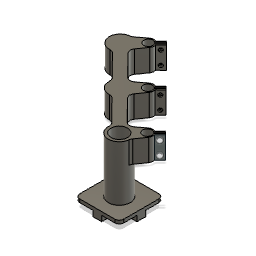
splicer_sample-fixation_004 (Autodesk Fusion 360 design; units mm, degrees)
Autodesk Fusion 360 part; units mm, degrees
sketch "Sketch1" plane through (0, 0, 0) normal (0, 1, 0) x (1, 0, 0)
  line L0 (20, -20) -> (-20, -20)
  line L1 (-20, -20) -> (-20, 20)
  line L2 (-20, 20) -> (20, 20)
  line L3 (20, 20) -> (20, -20)
  line L4 (20, -20) -> (-20, 20) construction
  line L5 (-20, -20) -> (20, 20) construction
  line L6 (-20, 4) -> (-15, 4)
  line L7 (-15, 4) -> (-15, -4)
  line L8 (-15, -4) -> (-20, -4)
  line L9 (-20, -4) -> (-20, 4)
  line L10 (-4, 20) -> (4, 20)
  line L11 (4, 20) -> (4, 15)
  line L12 (4, 15) -> (-4, 15)
  line L13 (-4, 15) -> (-4, 20)
  line L14 (20, 4) -> (15, 4)
  line L15 (15, 4) -> (15, -4)
  line L16 (15, -4) -> (20, -4)
  line L17 (20, -4) -> (20, 4)
  line L18 (-4, -20) -> (4, -20)
  line L19 (4, -20) -> (4, -15)
  line L20 (4, -15) -> (-4, -15)
  line L21 (-4, -15) -> (-4, -20)
  dimension "d1" = 40
  dimension "d2" = 40
  dimension "d3" = 5
  dimension "d4" = 8
  dimension "d5" = 16
  dimension "d6" = 5
  dimension "d7" = 16
  dimension "d8" = 8
  dimension "d9" = 5
  dimension "d10" = 5
  dimension "d11" = 8
  dimension "d12" = 8
  dimension "d13" = 16
  dimension "d14" = 16
  constraint horizontal L0
  constraint perpendicular L0 L1
  constraint parallel L0 L2
  constraint parallel L1 L3
  constraint coincident L4 origin
  constraint coincident L5 origin
  constraint horizontal L6
  constraint vertical L7
  constraint horizontal L8
  constraint vertical L9
  constraint coincident L1 L6.start
  constraint horizontal L10
  constraint vertical L11
  constraint horizontal L12
  constraint vertical L13
  constraint coincident L2 L10.start
  constraint horizontal L14
  constraint vertical L15
  constraint horizontal L16
  constraint vertical L17
  constraint coincident L3 L14.start
  constraint horizontal L18
  constraint vertical L19
  constraint horizontal L20
  constraint vertical L21
  constraint coincident L0 L18.start
  measures "d1" distance of L1.end L2.end
  measures "d2" distance of L0.end L1.end
  measures "d3" distance of L6.start L6.end
  measures "d4" distance of L6.start L8.end
  measures "d5" distance of L1.end L6.start
  measures "d6" distance of L10.start L12.end
  measures "d7" distance of L1.end L10.start
  measures "d8" distance of L11 L13
  measures "d9" distance of L18.start L20.end
  measures "d10" distance of L14.start L14.end
  measures "d11" distance of L14.end L15.end
  measures "d12" distance of L19.end L20.end
  measures "d13" distance of L1 L21
  measures "d14" distance of L0.start L16
extrude "Extrude1" add sketch "Sketch1" against normal blind 3 contours L0 L1 L2 L3 L6 L7 L8 L11 L12 L13 L14 L15 L16 L19 L20 L21 makes body 1
extrude "Extrude2" add sketch "Sketch1" against normal blind 8 contours L0 L18 L19 L20 L21 | L3 L14 L15 L16 L17 | L1 L6 L7 L8 L9 | L2 L10 L11 L12 L13 bodies 1
hole "Hole1" at (0, 0, 0) direction (0, -1, 0) diameter 9 depth 30 tip angle 118 bodies 1
fillet "Fillet1" radius 4 4 edges at (20, -1.5, -20) (-20, -1.5, -20) (20, -1.5, 20) (-20, -1.5, 20) on bodies 1
sketch "Sketch2" plane through (0, 0, 0) normal (0, 1, 0) x (1, 0, 0)
  circle A0 centre (0, 0) radius 10
  dimension "d24" = 20
  constraint coincident A0.centre origin
  measures "d24" diameter of A0
extrude "Extrude3" add sketch "Sketch2" along normal blind 50 bodies 1
sketch "Sketch3" plane through (0, 50, 0) normal (0, 1, 0) x (-1, 0, 0)
  circle A0 centre (0, 0) radius 10
hole "Hole2" at (0, 50, 0) direction (0, -1, 0) diameter 9 depth 90 tip angle 118 counterbore diameter 15 counterbore depth 45 bodies 1
sketch "Sketch4" plane through (0, 50, 0) normal (0, 1, 0) x (-1, 0, 0)
  circle A0 centre (0, 0) radius 7.5
  circle A1 centre (0, 0) radius 10
  circle A2 centre (-12.5974, -12.8571) radius 4.2
  circle A3 centre (-12.5974, -12.8571) radius 5.2
  line L0 (-9.9991, -0.1315) -> (-16.8496, -9.8641)
  line L1 (-0.1344, -9.9991) -> (-9.4743, -17.0148)
  line L2 (-14.7075, -17.3177) -> (-17.5526, -14.4336)
  line L3 (-17.5526, -14.4336) -> (-22.562, -19.3755)
  line L4 (-22.562, -19.3755) -> (-19.7168, -22.2595)
  line L5 (-19.7168, -22.2595) -> (-14.7075, -17.3177)
  dimension "d32" = 8.4
  dimension "d33" = 18
  dimension "d34" = 12.8571
  dimension "d35" = 1
  constraint coincident A1 L0.start
  constraint coincident A3 L0.end
  constraint tangent A3 L0
  constraint coincident A1 L1.start
  constraint coincident A3 L1.end
  constraint tangent A3 L1
  constraint perpendicular L2 L3
  constraint parallel L2 L4
  constraint parallel L3 L5
  constraint coincident A3 L2.end
  measures "d32" diameter of A2
  measures "d33" distance of A0.centre A2.centre
  measures "d34" vertical distance of A0.centre A2.centre
extrude "Extrude4" add sketch "Sketch4" against normal blind 20 separate body contours A1 A3 L0 L1 | A3 L2 L5 | A3 L2 L5 | A3 L3 L4 L5 makes body 2
sketch "Sketch5" plane through (0, 50, 0) normal (0, 1, 0) x (-1, 0, 0)
  circle A0 centre (-12.5974, -12.8571) radius 4.2
  line L0 (-9.9991, -0.1315) -> (-16.8496, -9.8641)
  arc A1 (-16.8496, -9.8641) -> (-17.5526, -14.4336) centre (-12.5974, -12.8571) ccw
  line L1 (-17.5526, -14.4336) -> (-22.562, -19.3755)
  line L2 (-22.562, -19.3755) -> (-19.7168, -22.2595)
  line L3 (-19.7168, -22.2595) -> (-14.908, -17.5156)
  arc A2 (-14.908, -17.5156) -> (-9.4743, -17.0148) centre (-12.5974, -12.8571) ccw
  line L4 (-9.4743, -17.0148) -> (-0.1344, -9.9991)
  arc A3 (-9.9991, -0.1315) -> (-0.1344, -9.9991) centre (0, 0) ccw
  line L5 (-20.5087, -21.4569) -> (-21.5424, -20.409)
  line L6 (-21.5424, -20.409) -> (-15.0226, -13.9771)
  line L7 (-15.0226, -13.9771) -> (-13.9888, -15.025)
  line L8 (-13.9888, -15.025) -> (-20.5087, -21.4569)
  constraint perpendicular L5 L6
  constraint parallel L5 L7
  constraint parallel L6 L8
  constraint coincident L2 L5.end
  constraint coincident L2 L5.start
extrude "Extrude5" cut sketch "Sketch5" against normal blind 20 contours A0 L2 L5 L6 L8 bodies 2
sketch "Sketch6" plane through (1.441, 0, 1.4607) normal (0.70229, 0, 0.711891) x (0.711891, 0, -0.70229)
  line L0 (29.6689, 50) -> (22.6322, 50)
  line L1 (22.6322, 50) -> (22.6322, 30)
  line L2 (22.6322, 30) -> (29.6689, 30)
  line L3 (29.6689, 30) -> (29.6689, 50)
  point P0 (26, 46)
  point P1 (26, 34)
hole "Hole3" at (19.9502, 46, -16.7988) at (19.9502, 34, -16.7988) direction (-0.70229, 0, -0.711891) diameter 2.93 depth 5 tip angle 118 bodies 2
thread "Thread1" "ISO Metric profile 3.5 M3.5x0.6 6H" thread offset 0 thread depth 10
hole "Hole4" at (19.9502, 46, -16.7988) at (19.9502, 34, -16.7988) direction (-0.70229, 0, -0.711891) diameter 3.4 depth 2 tip angle 118 bodies 2
pattern_linear "R-Pattern1" count 3 spacing 50 along (-0.70229, 0, -0.711891) of bodies 2 makes body 3 at (-18.3529, 43.3333, -47.9044) makes body 4 at (-60.9846, 43.3333, -86.5756)
sketch "Sketch7" plane through (0, 50, 0) normal (0, 1, 0) x (-1, 0, 0)
  line L0 (13.5721, -56.0036) -> (18.9614, -50.687)
  arc A0 (19.952, -51.7774) -> (18.9614, -50.687) centre (22.5171, -48.4517) ccw
  line L1 (19.952, -51.7774) -> (14.6058, -57.0515)
  line L2 (14.6058, -57.0515) -> (15.3977, -57.8541)
  line L3 (15.3977, -57.8541) -> (20.2065, -53.1101)
  arc A1 (20.2065, -53.1101) -> (25.6402, -52.6094) centre (22.5171, -48.4517) ccw
  line L4 (25.6402, -52.6094) -> (34.9801, -45.5936)
  arc A2 (25.1154, -35.726) -> (34.9801, -45.5936) centre (35.1145, -35.5945) ccw
  line L5 (25.1154, -35.726) -> (18.2649, -45.4586)
  arc A3 (18.2649, -45.4586) -> (17.5619, -50.0282) centre (22.5171, -48.4517) ccw
  line L6 (17.5619, -50.0282) -> (12.5525, -54.97)
  line L7 (12.5525, -54.97) -> (13.5721, -56.0036)
  circle A4 centre (35.1145, -35.5945) radius 10
  arc A5 (60.2299, -71.3206) -> (70.0946, -81.1882) centre (70.229, -71.1891) ccw
  circle A6 centre (70.229, -71.1891) radius 10
  line L8 (0, 0) -> (70.229, -71.1891)
  line L9 (-3.5595, -3.5115) -> (66.6696, -74.7005)
  line L10 (3.5595, 3.5115) -> (73.7885, -67.6776)
  circle A7 centre (0, 0) radius 10
  dimension "d52" = 20
  dimension "d53" = 5
  dimension "d54" = -5
  constraint concentric A2 A4
  constraint concentric A5 A6
  constraint coincident L8.start A7.centre
  constraint coincident A5.centre A6.centre
  measures "d52" diameter of A4
extrude "Extrude6" add sketch "Sketch7" against normal blind 20 contours A2 A4 L9 | A4 L8 L9 A7 | A4 L8 L9 | A4 A6 L8 L9 | A4 L8 L10 A7 | A4 L8 L10 | A4 A6 L8 L10 | A5 A6 | A4 L10 bodies 1 3 4
combine "Combine2" operation add target body 1 tool bodies 2
fillet "Fillet2" radius 5 14 edges at (-9.6415, 40, -2.6537) (-32.5919, 40, -25.9179) (-44.756, 40, -38.2483) (-67.7065, 40, -61.5125) (-70.0946, 40, -81.1882) (-34.9801, 40, -45.5936) (-37.6371, 40, -45.2712) (-2.5226, 40, -9.6766) (-25.473, 40, -32.9408) (-25.1154, 40, -35.726) (-60.2299, 40, -71.3206) (-60.5875, 40, -68.5354) (0.1344, 40, -9.9991) (9.9991, 40, -0.1315) on bodies 1
pattern_circular "C-Pattern1" [suppressed]
combine "Combine1" [suppressed]
equation "d6 = d3"
equation "d7 = d5"
equation "d8 = d4"
equation "d9 = d3"
equation "d10 = d3"
equation "d11 = d4"
equation "d12 = d4"
equation "d13 = d7"
equation "d14 = d7"
equation "d34 = d33 / 1.4"
named bodies: "4040_fixation_base"
